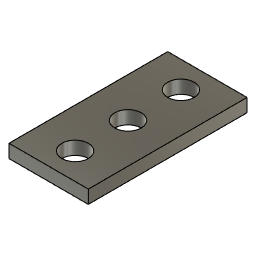
base+2 (Autodesk Fusion 360 design; units mm, degrees)
Autodesk Fusion 360 part; units mm, degrees
box "Primitiva de caixa1" add length 60 width 30 height 5 placed x (0, 1, 0) y (-1, 0, 0) z (0, 0, 1) at (30, 0, 0)
cylinder "Cilindro primitivo1" cut diameter 10 height -42 placed x (1, 0, 0) y (0, 1, 0) z (0, 0, 1) at (15, 10, 5)
cylinder "Cilindro primitivo2" cut diameter 10 height -21 placed x (1, 0, 0) y (0, 1, 0) z (0, 0, 1) at (15, 50, 5)
cylinder "Cilindro primitivo3" cut diameter 10 height -17 placed x (1, 0, 0) y (0, 1, 0) z (0, 0, 1) at (15, 30, 5)
